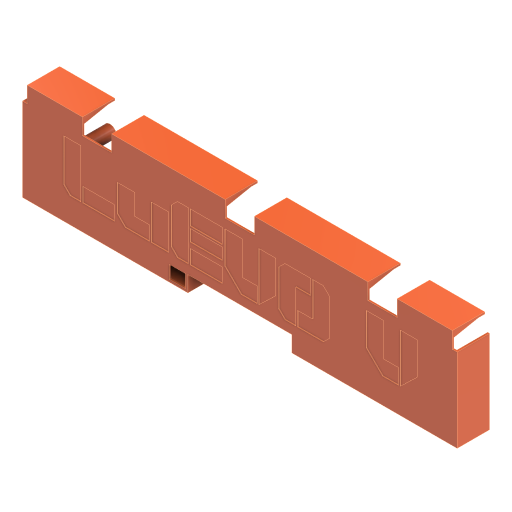
# Autodesk Inventor part: WiringCover
Saved by Autodesk Inventor 2023.2 (Build 272271000, 271)
## iProperties
Created: 2023-02-27
Part Number: WiringCover
Material: ABS Plastic
Document SubType Name: Modeling
Designer: remop
Density: 1.06 g/cm^3
Appearance: Smooth - Light Orange
Author: remop
Autodesk Inventor part; units mm, degrees
ref_plane "YZ Plane" through (0, 0, 0) normal (1, 0, 0) x (0, 1, 0)
ref_plane "XZ Plane" through (0, 0, 0) normal (0, 1, 0) x (-1, 0, 0)
ref_plane "XY Plane" through (0, 0, 0) normal (0, 0, 1) x (1, 0, 0)
sketch "Sketch1" plane through (0, 0, 0) normal (0, 0, 1) x (1, 0, 0)
  line L0 (-105.5, 113.5) -> (-109, 117) projected
  line L1 (-105.5, 113.5) -> (-70.5, 113.5) projected
  line L2 (-67, 117) -> (-70.5, 113.5) projected
  line L3 (-67, 117) -> (-67, 152) projected
  line L4 (-70.5, 155.5) -> (-67, 152) projected
  line L5 (-70.5, 155.5) -> (-105.5, 155.5) projected
  line L6 (-109, 152) -> (-105.5, 155.5) projected
  line L7 (-109, 152) -> (-109, 117) projected
  line L8 (-17.5, 113.5) -> (-21, 117) projected
  line L9 (-17.5, 113.5) -> (17.5, 113.5) projected
  line L10 (21, 117) -> (17.5, 113.5) projected
  line L11 (21, 117) -> (21, 152) projected
  line L12 (17.5, 155.5) -> (21, 152) projected
  line L13 (17.5, 155.5) -> (-17.5, 155.5) projected
  line L14 (-21, 152) -> (-17.5, 155.5) projected
  line L15 (-21, 152) -> (-21, 117) projected
  line L16 (70.5, 113.5) -> (67, 117) projected
  line L17 (70.5, 113.5) -> (105.5, 113.5) projected
  line L18 (109, 117) -> (105.5, 113.5) projected
  line L19 (109, 117) -> (109, 152) projected
  line L20 (105.5, 155.5) -> (109, 152) projected
  line L21 (105.5, 155.5) -> (70.5, 155.5) projected
  line L22 (67, 152) -> (70.5, 155.5) projected
  line L23 (67, 152) -> (67, 117) projected
  circle A0 centre (25, 54.5) radius 1.45 projected
  circle A1 centre (-25, 54.5) radius 1.45 projected
  line L24 (31, 58.9018) -> (31, 50.0982) projected
  line L25 (31, 50.0982) -> (-31, 50.0982) projected
  line L26 (-31, 58.9018) -> (-31, 50.0982) projected
  line L27 (31, 58.9018) -> (-31, 58.9018) projected
  line L28 (134, 111.5) -> (-134, 111.5)
  line L29 (-134, 111.5) -> (-134, 50.0982)
  line L30 (-134, 50.0982) -> (-32, 50.0982)
  line L31 (-32, 50.0982) -> (-32, 59.9018)
  line L32 (-32, 59.9018) -> (32, 59.9018)
  line L33 (32, 59.9018) -> (32, 50.0982)
  line L34 (32, 50.0982) -> (134, 50.0982)
  line L35 (134, 50.0982) -> (134, 111.5)
  point P0 (0, 0)
  dimension "d0" = 25
  dimension "d1" = 25
  dimension "d2" = 2
  dimension "d3" = 268
  dimension "d4" = 1
  dimension "d5" = 1
  dimension "d6" = 1
  constraints: 16 end point, 5 perpendicular, 2 point on line, 1 horizontal, 1 horizontal alignment, 1 vertical
  measures "d0" distance from line of L28.end L7
  measures "d1" distance from line of L28.start L19
  measures "d2" distance between parallel lines of L28 L1
  measures "d3" distance of L28.start L28.end
  measures "d4" distance between parallel lines of L27 L32
  measures "d5" distance between parallel lines of L24 L33
  measures "d6" distance between parallel lines of L31 L26
extrude "Extrusion1" add sketch "Sketch1" along normal blind 20 contours L35 L34 L33 L32 L31 L30 L29 L28
sketch "Sketch2" plane through (0, 0, 0) normal (0, 0, -1) x (-1, 0, 0)
  line L0 (134, 111.5) -> (134, 50.0982) projected
  line L1 (-134, 111.5) -> (134, 111.5) projected
  line L2 (-134, 50.0982) -> (-134, 111.5) projected
  line L3 (-32, 50.0982) -> (-134, 50.0982) projected
  line L4 (-32, 59.9018) -> (-32, 50.0982) projected
  line L5 (32, 59.9018) -> (-32, 59.9018) projected
  line L6 (32, 50.0982) -> (32, 59.9018) projected
  line L7 (134, 50.0982) -> (32, 50.0982) projected
  line L8 (132.8, 110.3) -> (132.8, 51.2982)
  line L9 (132.8, 51.2982) -> (33.2, 51.2982)
  line L10 (33.2, 51.2982) -> (33.2, 61.1018)
  line L11 (33.2, 61.1018) -> (-33.2, 61.1018)
  line L12 (-33.2, 61.1018) -> (-33.2, 51.2982)
  line L13 (-33.2, 51.2982) -> (-132.8, 51.2982)
  line L14 (-132.8, 51.2982) -> (-132.8, 110.3)
  line L15 (-132.8, 110.3) -> (132.8, 110.3)
  point P0 (0, 0)
  dimension "d9" = 1.2
  constraints: 16 end point, 7 other
  measures "d9" distance between parallel lines of L1 L15
extrude "Extrusion2" cut sketch "Sketch2" against normal blind 19 contours L8 L9 L10 L11 L12 L13 L14 L15
sketch "Sketch3" plane through (0, 0, 20) normal (0, 0, 1) x (1, 0, 0)
  line L0 (-134, 111.5) -> (-134, 50.0982) projected
  line L1 (-134, 50.0982) -> (-32, 50.0982) projected
  line L2 (-32, 50.0982) -> (-32, 59.9018) projected
  line L3 (-32, 59.9018) -> (32, 59.9018) projected
  line L4 (32, 59.9018) -> (32, 50.0982) projected
  line L5 (32, 50.0982) -> (134, 50.0982) projected
  line L6 (134, 50.0982) -> (134, 111.5) projected
  line L7 (134, 111.5) -> (-134, 111.5) projected
  line L8 (-33.5, 51.5982) -> (-43.5, 51.5982)
  line L9 (-43.5, 51.5982) -> (-43.5, 59.5982)
  line L10 (-43.5, 59.5982) -> (-33.5, 59.5982)
  line L11 (-33.5, 59.5982) -> (-33.5, 51.5982)
  line L12 (134, 111.5) -> (-134, 111.5) projected
  line L13 (9, 101.5) -> (-9, 101.5)
  line L14 (-9, 101.5) -> (-9, 111.5)
  line L15 (-9, 111.5) -> (9, 111.5)
  line L16 (9, 111.5) -> (9, 101.5)
  line L17 (9, 101.5) -> (-9, 111.5) construction
  line L18 (-9, 101.5) -> (9, 111.5) construction
  line L19 (-97, 101.5) -> (-79, 101.5)
  line L20 (-79, 101.5) -> (-79, 111.5)
  line L21 (-79, 111.5) -> (-97, 111.5)
  line L22 (-97, 111.5) -> (-97, 101.5)
  line L23 (-97, 101.5) -> (-79, 111.5) construction
  line L24 (-79, 101.5) -> (-97, 111.5) construction
  line L25 (97, 101.5) -> (79, 101.5)
  line L26 (79, 101.5) -> (79, 111.5)
  line L27 (79, 111.5) -> (97, 111.5)
  line L28 (97, 111.5) -> (97, 101.5)
  line L29 (97, 101.5) -> (79, 111.5) construction
  line L30 (79, 101.5) -> (97, 111.5) construction
  line L31 (-131, 111.5) -> (-134, 111.5)
  line L32 (-134, 111.5) -> (-134, 101.5)
  line L33 (-134, 101.5) -> (-131, 101.5)
  line L34 (-131, 101.5) -> (-131, 111.5)
  line L35 (131, 111.5) -> (134, 111.5)
  line L36 (134, 111.5) -> (134, 101.5)
  line L37 (134, 101.5) -> (131, 101.5)
  line L38 (131, 101.5) -> (131, 111.5)
  point P0 (0, 0)
  point P1 (-33.5, 55.5982)
  point P2 (0, 106.5)
  point P3 (-88, 106.5)
  point P4 (88, 106.5)
  point P5 (9, 111.5)
  point P6 (-9, 111.5)
  point P7 (-97, 111.5)
  point P8 (0, 59.9018)
  dimension "d12" = 1.5
  dimension "d13" = 1.5
  dimension "d14" = 10
  dimension "d15" = 8
  dimension "d18" = 18
  dimension "d19" = 10
  dimension "d25" = 3
  dimension "d26" = 88
  dimension "d27" = 88
  constraints: 60 end point, 12 parallel, 8 midpoint, 7 equal length, 7 point on line, 6 horizontal, 6 perpendicular, 1 vertical alignment
  measures "d12" distance from line of L2 point (-33.5, 55.598)
  measures "d13" distance between parallel lines of L1 L8
  measures "d14" distance of L8.start L8.end
  measures "d15" distance of L8.end L9.end
  measures "d18" distance of L13.start L13.end
  measures "d19" distance of L15.end L13.start
  measures "d25" distance of L32.end L33.end
  measures "d26" distance of point (0, 106.5) point (-88, 106.5)
  measures "d27" distance of point (88, 106.5) point (0, 106.5)
extrude "Extrusion3" cut sketch "Sketch3" against normal through all contours L7 L34 L33 L0 | L7 L20 L19 L22 | L7 L16 L13 L14 | L7 L28 L25 L26 | L37 L38 L7 L6 | L8 L9 L10 L11
sketch "Sketch4" plane through (-134, 50.0982, 0) normal (-1, 0, 0) x (0, 0, 1)
  line L0 (0, 51.4018) -> (0, 0) projected
  line L1 (0, 0) -> (20, 0) projected
  line L2 (20, 51.4018) -> (20, 0) projected
  line L3 (0, 9.8036) -> (0, 0) projected
  line L4 (0, 5) -> (10, 5)
  line L5 (10, 5) -> (10, 25)
  line L6 (10, 25) -> (0, 25)
  line L7 (0, 25) -> (0, 5)
  line L8 (20, 51.4018) -> (0, 51.4018) projected
  point P0 (0, -50.0982)
  point P1 (0, 25)
  dimension "d20" = 5
  dimension "d21" = 20
  dimension "d22" = 10
  constraints: 8 end point, 2 parallel, 1 horizontal, 1 perpendicular, 1 point on line
  measures "d20" distance between parallel lines of L1 L4
  measures "d21" distance of L4.end L5.end
  measures "d22" distance of L4.start L4.end
extrude "Extrusion4" cut sketch "Sketch4" against normal up to surface (55 mm away) contours L6 L5 L4 L0
chamfer "Chamfer1" distance 15 distance2 3 1 edges at (114, 110.3, 19) measured on face at (108.3333, 110.3, 6.3333)
chamfer "Chamfer2" distance 15 distance2 3 1 edges at (44, 110.3, 19) measured on face at (32.3333, 110.3, 6.3333)
chamfer "Chamfer3" distance 15 distance2 3 1 edges at (-44, 110.3, 19) measured on face at (-55.6667, 110.3, 6.3333)
chamfer "Chamfer4" distance 15 distance2 3 1 edges at (-114, 110.3, 19) measured on face at (-119.6667, 110.3, 12.6667)
sketch "Sketch6" plane through (0, 0, 20) normal (0, 0, 1) x (1, 0, 0)
  line L0 (-97, 101.5) -> (-97, 111.5) projected
  line L1 (-97, 111.5) -> (-131, 111.5) projected
  line L2 (-131, 111.5) -> (-131, 101.5) projected
  line L3 (-131, 101.5) -> (-134, 101.5) projected
  line L4 (-134, 101.5) -> (-134, 50.0982) projected
  line L5 (-134, 50.0982) -> (-32, 50.0982) projected
  line L6 (-32, 50.0982) -> (-32, 59.9018) projected
  line L7 (-32, 59.9018) -> (32, 59.9018) projected
  line L8 (32, 59.9018) -> (32, 50.0982) projected
  line L9 (32, 50.0982) -> (134, 50.0982) projected
  line L10 (134, 50.0982) -> (134, 101.5) projected
  line L11 (134, 101.5) -> (131, 101.5) projected
  line L12 (131, 101.5) -> (131, 111.5) projected
  line L13 (131, 111.5) -> (97, 111.5) projected
  line L14 (97, 111.5) -> (97, 101.5) projected
  line L15 (97, 101.5) -> (79, 101.5) projected
  line L16 (79, 101.5) -> (79, 111.5) projected
  line L17 (79, 111.5) -> (9, 111.5) projected
  line L18 (9, 111.5) -> (9, 101.5) projected
  line L19 (9, 101.5) -> (-9, 101.5) projected
  line L20 (-9, 101.5) -> (-9, 111.5) projected
  line L21 (-9, 111.5) -> (-79, 111.5) projected
  line L22 (-79, 111.5) -> (-79, 101.5) projected
  line L23 (-79, 101.5) -> (-97, 101.5) projected
  line L24 (-43.5, 51.5982) -> (-43.5, 59.5982) projected
  line L25 (-43.5, 59.5982) -> (-33.5, 59.5982) projected
  line L26 (-33.5, 59.5982) -> (-33.5, 51.5982) projected
  line L27 (-33.5, 51.5982) -> (-43.5, 51.5982) projected
  line L28 (-134, 101.5) -> (134, 101.5) construction
  line L29 (134, 101.5) -> (134, 59.9018) construction
  line L30 (134, 59.9018) -> (-134, 59.9018) construction
  line L31 (-134, 59.9018) -> (-134, 101.5) construction
  line L32 (-104.5991, 65.7147) -> (-108.4977, 69.6133)
  line L33 (-108.4977, 69.6133) -> (-108.4977, 95.7147)
  line L34 (-108.4977, 95.7147) -> (-98.0461, 95.7147)
  line L35 (-98.0461, 95.7147) -> (-98.0461, 65.7147)
  line L36 (-98.0461, 65.7147) -> (-104.5991, 65.7147)
  line L37 (-96.8295, 65.7147) -> (-96.8295, 74.5903)
  line L38 (-96.8295, 74.5903) -> (-77.1429, 74.5903)
  line L39 (-77.1429, 74.5903) -> (-77.1429, 65.7147)
  line L40 (-77.1429, 65.7147) -> (-96.8295, 65.7147)
  line L41 (-55.7143, 65.7424) -> (-70.6452, 65.7424)
  line L42 (-70.6452, 65.7424) -> (-75.4839, 70.5811)
  line L43 (-75.4839, 70.5811) -> (-75.4839, 87.3645)
  line L44 (-75.4839, 87.3645) -> (-64.894, 87.3645)
  line L45 (-64.894, 87.3645) -> (-64.894, 74.6179)
  line L46 (-64.894, 74.6179) -> (-55.7143, 74.6179)
  line L47 (-55.7143, 74.6179) -> (-55.7143, 65.7424)
  line L48 (-43.9631, 65.7424) -> (-54.553, 65.7424)
  line L49 (-54.553, 65.7424) -> (-54.553, 87.3645)
  line L50 (-54.553, 87.3645) -> (-43.9631, 87.3645)
  line L51 (-43.9631, 87.3645) -> (-43.9631, 65.7424)
  line L52 (-31.7696, 65.7147) -> (-38.4055, 65.7147)
  line L53 (-38.4055, 65.7147) -> (-42.3041, 69.6133)
  line L54 (-42.3041, 69.6133) -> (-42.3041, 91.8161)
  line L55 (-42.3041, 91.8161) -> (-38.4055, 95.7147)
  line L56 (-38.4055, 95.7147) -> (-31.7696, 95.7147)
  line L57 (-31.7696, 95.7147) -> (-31.7696, 65.7147)
  line L58 (-10.7834, 86.452) -> (-30.553, 86.452)
  line L59 (-30.553, 86.452) -> (-30.553, 95.7147)
  line L60 (-30.553, 95.7147) -> (-10.7834, 95.7147)
  line L61 (-10.7834, 95.7147) -> (-10.7834, 86.452)
  line L62 (-10.7834, 65.7147) -> (-30.553, 65.7147)
  line L63 (-30.553, 65.7147) -> (-30.553, 74.5903)
  line L64 (-30.553, 74.5903) -> (-10.7834, 74.5903)
  line L65 (-10.7834, 74.5903) -> (-10.7834, 65.7147)
  line L66 (-10.7834, 77.9636) -> (-30.553, 77.9636)
  line L67 (-30.553, 77.9636) -> (-30.553, 85.2355)
  line L68 (-30.553, 85.2355) -> (-10.7834, 85.2355)
  line L69 (-10.7834, 85.2355) -> (-10.7834, 77.9636)
  line L70 (10.6452, 65.6871) -> (0.8295, 65.6871)
  line L71 (0.8295, 65.6871) -> (-9.1244, 75.641)
  line L72 (-9.1244, 75.641) -> (-9.1244, 95.7147)
  line L73 (-9.1244, 95.7147) -> (1.4654, 95.7147)
  line L74 (1.4654, 95.7147) -> (1.4654, 75.1709)
  line L75 (1.4654, 75.1709) -> (10.6452, 75.1709)
  line L76 (10.6452, 75.1709) -> (10.6452, 65.6871)
  line L77 (11.8065, 65.7147) -> (11.8065, 95.7147)
  line L78 (11.8065, 95.7147) -> (22.2304, 95.7147)
  line L79 (22.2304, 95.7147) -> (22.2304, 75.6963)
  line L80 (22.2304, 75.6963) -> (11.8065, 65.7147)
  line L81 (34.4793, 65.7147) -> (27.788, 65.7147)
  line L82 (27.788, 65.7147) -> (23.8894, 69.6133)
  line L83 (23.8894, 69.6133) -> (23.8894, 91.8161)
  line L84 (23.8894, 91.8161) -> (27.8157, 95.7147)
  line L85 (27.8157, 95.7147) -> (43.659, 95.7147)
  line L86 (43.659, 95.7147) -> (43.659, 86.452)
  line L87 (43.659, 86.452) -> (34.4793, 86.452)
  line L88 (34.4793, 86.452) -> (34.4793, 65.7147)
  line L89 (55.4101, 69.641) -> (51.4839, 65.7147)
  line L90 (51.4839, 65.7147) -> (35.5853, 65.7147)
  line L91 (35.5853, 65.7147) -> (35.5853, 74.5903)
  line L92 (35.5853, 74.5903) -> (44.8203, 74.5903)
  line L93 (44.8203, 74.5903) -> (44.8203, 95.7147)
  line L94 (44.8203, 95.7147) -> (51.4839, 95.7147)
  line L95 (51.4839, 95.7147) -> (55.4101, 91.7884)
  line L96 (55.4101, 91.7884) -> (55.4101, 69.641)
  line L97 (97.7419, 65.6871) -> (87.9263, 65.6871)
  line L98 (87.9263, 65.6871) -> (77.9723, 75.641)
  line L99 (77.9723, 75.641) -> (77.9723, 95.7147)
  line L100 (77.9723, 95.7147) -> (88.5622, 95.7147)
  line L101 (88.5622, 95.7147) -> (88.5622, 75.1709)
  line L102 (88.5622, 75.1709) -> (97.7419, 75.1709)
  line L103 (97.7419, 75.1709) -> (97.7419, 65.6871)
  line L104 (98.9032, 65.7147) -> (98.9032, 95.7147)
  line L105 (98.9032, 95.7147) -> (109.3272, 95.7147)
  line L106 (109.3272, 95.7147) -> (109.3272, 75.6963)
  line L107 (109.3272, 75.6963) -> (98.9032, 65.7147)
  point P0 (0, 0)
  constraints: 2 coincident, 2 horizontal alignment, 2 other
extrude "Extrusion5" cut sketch "Sketch6" against normal blind 0.4 contours L32 L33 L34 L35 L36 | L37 L38 L39 L40 | L41 L42 L43 L44 L45 L46 L47 | L48 L49 L50 L51 | L52 L53 L54 L55 L56 L57 | L58 L59 L60 L61 | L62 L63 L64 L65 | L66 L67 L68 L69 | L70 L71 L72 L73 L74 L75 L76 | L77 L78 L79 L80 | L81 L82 L83 L84 L85 L86 L87 L88 | L89 L90 L91 L92 L93 L94 L95 L96 | L97 L98 L99 L100 L101 L102 L103 | L104 L105 L106 L107
sketch "Sketch7" plane through (0, 0, 19) normal (0, 0, -1) x (-1, 0, 0)
  line L0 (43.5, 59.5982) -> (43.5, 51.5982) projected
  line L1 (43.5, 51.5982) -> (33.5, 51.5982) projected
  line L2 (33.5, 51.5982) -> (33.5, 59.5982) projected
  line L3 (33.5, 59.5982) -> (43.5, 59.5982) projected
  line L4 (97, 107.3) -> (131, 107.3) projected
  line L5 (97, 107.3) -> (97, 101.5) projected
  line L6 (97, 101.5) -> (79, 101.5) projected
  line L7 (79, 101.5) -> (79, 107.3) projected
  line L8 (9, 107.3) -> (79, 107.3) projected
  line L9 (9, 107.3) -> (9, 101.5) projected
  line L10 (9, 101.5) -> (-9, 101.5) projected
  line L11 (-9, 101.5) -> (-9, 107.3) projected
  line L12 (-79, 107.3) -> (-9, 107.3) projected
  line L13 (-79, 107.3) -> (-79, 101.5) projected
  line L14 (-79, 101.5) -> (-97, 101.5) projected
  line L15 (-97, 101.5) -> (-97, 107.3) projected
  line L16 (-131, 107.3) -> (-97, 107.3) projected
  line L17 (-131, 107.3) -> (-131, 101.5) projected
  line L18 (-131, 101.5) -> (-132.8, 101.5) projected
  line L19 (-132.8, 51.2982) -> (-132.8, 101.5) projected
  line L20 (-33.2, 51.2982) -> (-132.8, 51.2982) projected
  line L21 (-33.2, 61.1018) -> (-33.2, 51.2982) projected
  line L22 (33.2, 61.1018) -> (-33.2, 61.1018) projected
  line L23 (33.2, 51.2982) -> (33.2, 61.1018) projected
  line L24 (132.8, 51.2982) -> (33.2, 51.2982) projected
  line L25 (132.8, 101.5) -> (132.8, 51.2982) projected
  line L26 (132.8, 101.5) -> (131, 101.5) projected
  line L27 (131, 101.5) -> (131, 107.3) projected
  circle A0 centre (100, 92.3) radius 1.4
  circle A1 centre (100, 92.3) radius 4
  circle A2 centre (100, 62.3) radius 1.4
  circle A3 centre (100, 62.3) radius 4
  circle A4 centre (-100, 92.3) radius 1.4
  circle A5 centre (-100, 92.3) radius 4
  circle A6 centre (-100, 62.3) radius 1.4
  circle A7 centre (-100, 62.3) radius 4
  point P0 (0, 0)
  point P1 (0, 101.5)
  dimension "d42" = 2.8
  dimension "d43" = 8
  dimension "d46" = 30
  dimension "d49" = 200
  dimension "d52" = 100
  dimension "d53" = 15
  constraints: 8 centre point, 4 coincident, 1 horizontal, 1 midpoint, 1 vertical, 12 other
  measures "d42" diameter of A0
  measures "d43" diameter of A1
  measures "d46" distance of A1.centre A3.centre
  measures "d49" distance of A1.centre A5.centre
  measures "d52" horizontal distance of A4.centre point (0, 101.5)
  measures "d53" distance from line of L16 A5.centre
extrude "Extrusion6" add sketch "Sketch7" along normal up to surface (19 mm away) contours A1 | A3 | A5 | A7
equation "\"d1\" = d0"
equation "\"d5\" = d4"
equation "\"d6\" = d4"
equation "\"d13\" = d12"
equation "\"d27\" = d26"
equation "\"d52\" = 0.5 * d49"
body "Solid1"
